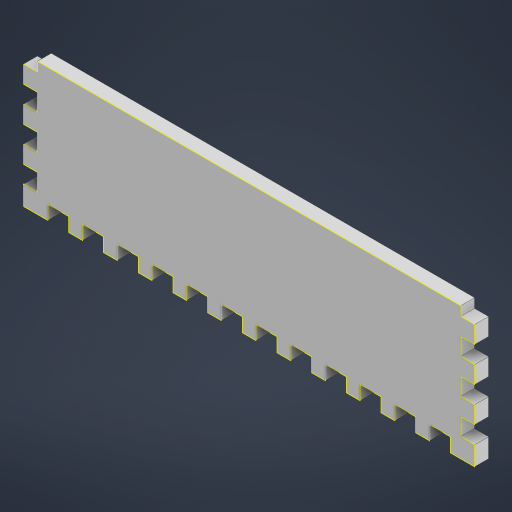
# Autodesk Inventor part: VorderWand
Saved by Autodesk Inventor 2023 (Build 270158030, 158C)
## iProperties
Created: 2022-06-21
Part Number: VorderWand
Material: Generic
Document SubType Name: Modeling
Designer: Simon
Density: 1 g/cm^3
Appearance: Default
Author: Simon
Autodesk Inventor part; units mm, degrees
ref_plane "YZ Plane" through (0, 0, 0) normal (1, 0, 0) x (0, 1, 0)
ref_plane "XZ Plane" through (0, 0, 0) normal (0, 1, 0) x (-1, 0, 0)
ref_plane "XY Plane" through (0, 0, 0) normal (0, 0, 1) x (1, 0, 0)
sketch "Sketch1" plane through (0, 0, 0) normal (0, 0, 1) x (1, 0, 0)
  line L0 (0, -5.5) -> (4, -5.5)
  line L1 (7, -5.5) -> (4, -5.5)
  line L2 (0, -5.5) -> (0, 0)
  line L3 (0, 0) -> (4, 0)
  line L4 (4, 5) -> (4, 0)
  line L5 (0, 5) -> (4, 5)
  line L6 (0, 5) -> (0, 10)
  line L7 (0, 10) -> (4, 10)
  line L8 (4, 15) -> (4, 10)
  line L9 (0, 15) -> (4, 15)
  line L10 (0, 15) -> (0, 20)
  line L11 (0, 20) -> (4, 20)
  line L12 (4, 25) -> (4, 20)
  line L13 (0, 25) -> (4, 25)
  line L14 (0, 25) -> (0, 30)
  line L15 (0, 30) -> (4, 30)
  line L16 (4, 32.6906) -> (4, 30)
  line L17 (7, -1.5) -> (7, -5.5)
  line L18 (7, -1.5) -> (13, -1.5)
  line L19 (13, -5.5) -> (13, -1.5)
  line L20 (17, -5.5) -> (13, -5.5)
  line L21 (17, -1.5) -> (17, -5.5)
  line L22 (17, -1.5) -> (23, -1.5)
  line L23 (23, -5.5) -> (23, -1.5)
  line L24 (27, -5.5) -> (23, -5.5)
  line L25 (27, -1.5) -> (27, -5.5)
  line L26 (27, -1.5) -> (33, -1.5)
  line L27 (33, -5.5) -> (33, -1.5)
  line L28 (37, -5.5) -> (33, -5.5)
  line L29 (37, -1.5) -> (37, -5.5)
  line L30 (37, -1.5) -> (43, -1.5)
  line L31 (43, -5.5) -> (43, -1.5)
  line L32 (47, -5.5) -> (43, -5.5)
  line L33 (47, -1.5) -> (47, -5.5)
  line L34 (47, -1.5) -> (53, -1.5)
  line L35 (53, -5.5) -> (53, -1.5)
  line L36 (57, -5.5) -> (53, -5.5)
  line L37 (57, -1.5) -> (57, -5.5)
  line L38 (57, -1.5) -> (63, -1.5)
  line L39 (63, -5.5) -> (63, -1.5)
  line L40 (67, -5.5) -> (63, -5.5)
  line L41 (67, -1.5) -> (67, -5.5)
  line L42 (67, -1.5) -> (73, -1.5)
  line L43 (73, -5.5) -> (73, -1.5)
  line L44 (77, -5.5) -> (73, -5.5)
  line L45 (77, -1.5) -> (77, -5.5)
  line L46 (77, -1.5) -> (83, -1.5)
  line L47 (83, -5.5) -> (83, -1.5)
  line L48 (87, -5.5) -> (83, -5.5)
  line L49 (87, -1.5) -> (87, -5.5)
  line L50 (87, -1.5) -> (93, -1.5)
  line L51 (93, -5.5) -> (93, -1.5)
  line L52 (97, -5.5) -> (93, -5.5)
  line L53 (97, -1.5) -> (97, -5.5)
  line L54 (97, -1.5) -> (103, -1.5)
  line L55 (103, -5.5) -> (103, -1.5)
  line L56 (107, -5.5) -> (103, -5.5)
  line L57 (107, -1.5) -> (107, -5.5)
  line L58 (107, -1.5) -> (113, -1.5)
  line L59 (113, -5.5) -> (113, -1.5)
  line L60 (117, -5.5) -> (113, -5.5)
  line L61 (117, -1.5) -> (117, -5.5)
  line L62 (117, -1.5) -> (123, -1.5)
  line L63 (123, -5.5) -> (123, -1.5)
  line L64 (126, -5.5) -> (123, -5.5)
  line L65 (126, -5.5) -> (130, -5.5)
  line L66 (130, 0) -> (130, -5.5)
  line L67 (130, 0) -> (126, 0)
  line L68 (126, 0) -> (126, 5)
  line L69 (126, 5) -> (130, 5)
  line L70 (130, 10) -> (130, 5)
  line L71 (126, 10) -> (130, 10)
  line L72 (126, 10) -> (126, 15)
  line L73 (126, 15) -> (130, 15)
  line L74 (130, 20) -> (130, 15)
  line L75 (126, 20) -> (130, 20)
  line L76 (126, 20) -> (126, 25)
  line L77 (126, 25) -> (130, 25)
  line L78 (130, 30) -> (130, 25)
  line L79 (126, 30) -> (130, 30)
  line L80 (126, 30) -> (126, 32.6906)
  line L81 (4, 32.6906) -> (126, 32.6906)
  point P0 (0, 0)
  constraints: 164 end point, 8 vertical, 1 horizontal, 8 other
extrude "Extrusion1" add sketch "Sketch1" along normal blind 4
sketch "Sketch2" plane through (0, 0, 4) normal (0, 0, 1) x (1, 0, 0)
  line L0 (0, -5.5) -> (7, -5.5) projected
  line L1 (7, -5.5) -> (7, -1.5) projected
  line L2 (7, -1.5) -> (13, -1.5) projected
  line L3 (13, -1.5) -> (13, -5.5) projected
  line L4 (13, -5.5) -> (17, -5.5) projected
  line L5 (17, -5.5) -> (17, -1.5) projected
  line L6 (17, -1.5) -> (23, -1.5) projected
  line L7 (23, -1.5) -> (23, -5.5) projected
  line L8 (23, -5.5) -> (27, -5.5) projected
  line L9 (27, -5.5) -> (27, -1.5) projected
  line L10 (27, -1.5) -> (33, -1.5) projected
  line L11 (33, -1.5) -> (33, -5.5) projected
  line L12 (33, -5.5) -> (37, -5.5) projected
  line L13 (37, -5.5) -> (37, -1.5) projected
  line L14 (37, -1.5) -> (43, -1.5) projected
  line L15 (43, -1.5) -> (43, -5.5) projected
  line L16 (43, -5.5) -> (47, -5.5) projected
  line L17 (47, -5.5) -> (47, -1.5) projected
  line L18 (47, -1.5) -> (53, -1.5) projected
  line L19 (53, -1.5) -> (53, -5.5) projected
  line L20 (53, -5.5) -> (57, -5.5) projected
  line L21 (57, -5.5) -> (57, -1.5) projected
  line L22 (57, -1.5) -> (63, -1.5) projected
  line L23 (63, -1.5) -> (63, -5.5) projected
  line L24 (63, -5.5) -> (67, -5.5) projected
  line L25 (67, -5.5) -> (67, -1.5) projected
  line L26 (67, -1.5) -> (73, -1.5) projected
  line L27 (73, -1.5) -> (73, -5.5) projected
  line L28 (73, -5.5) -> (77, -5.5) projected
  line L29 (77, -5.5) -> (77, -1.5) projected
  line L30 (77, -1.5) -> (83, -1.5) projected
  line L31 (83, -1.5) -> (83, -5.5) projected
  line L32 (83, -5.5) -> (87, -5.5) projected
  line L33 (87, -5.5) -> (87, -1.5) projected
  line L34 (87, -1.5) -> (93, -1.5) projected
  line L35 (93, -1.5) -> (93, -5.5) projected
  line L36 (93, -5.5) -> (97, -5.5) projected
  line L37 (97, -5.5) -> (97, -1.5) projected
  line L38 (97, -1.5) -> (103, -1.5) projected
  line L39 (103, -1.5) -> (103, -5.5) projected
  line L40 (103, -5.5) -> (107, -5.5) projected
  line L41 (107, -5.5) -> (107, -1.5) projected
  line L42 (107, -1.5) -> (113, -1.5) projected
  line L43 (113, -1.5) -> (113, -5.5) projected
  line L44 (113, -5.5) -> (117, -5.5) projected
  line L45 (117, -5.5) -> (117, -1.5) projected
  line L46 (117, -1.5) -> (123, -1.5) projected
  line L47 (123, -1.5) -> (123, -5.5) projected
  line L48 (123, -5.5) -> (130, -5.5) projected
  line L49 (130, -5.5) -> (130, 0) projected
  line L50 (130, 0) -> (126, 0) projected
  line L51 (126, 0) -> (126, 5) projected
  line L52 (126, 5) -> (130, 5) projected
  line L53 (130, 5) -> (130, 10) projected
  line L54 (130, 10) -> (126, 10) projected
  line L55 (126, 10) -> (126, 15) projected
  line L56 (126, 15) -> (130, 15) projected
  line L57 (130, 15) -> (130, 20) projected
  line L58 (130, 20) -> (126, 20) projected
  line L59 (126, 20) -> (126, 25) projected
  line L60 (126, 25) -> (130, 25) projected
  line L61 (130, 25) -> (130, 30) projected
  line L62 (130, 30) -> (126, 30) projected
  line L63 (126, 30) -> (126, 32.6906) projected
  line L64 (126, 32.6906) -> (4, 32.6906) projected
  line L65 (4, 32.6906) -> (4, 30) projected
  line L66 (4, 30) -> (0, 30) projected
  line L67 (0, 30) -> (0, 25) projected
  line L68 (0, 25) -> (4, 25) projected
  line L69 (4, 25) -> (4, 20) projected
  line L70 (4, 20) -> (0, 20) projected
  line L71 (0, 20) -> (0, 15) projected
  line L72 (0, 15) -> (4, 15) projected
  line L73 (4, 15) -> (4, 10) projected
  line L74 (4, 10) -> (0, 10) projected
  line L75 (0, 10) -> (0, 5) projected
  line L76 (0, 5) -> (4, 5) projected
  line L77 (4, 5) -> (4, 0) projected
  line L78 (4, 0) -> (0, 0) projected
  line L79 (0, 0) -> (0, -5.5) projected
  point P0 (0, 0)
body "Solid1"
